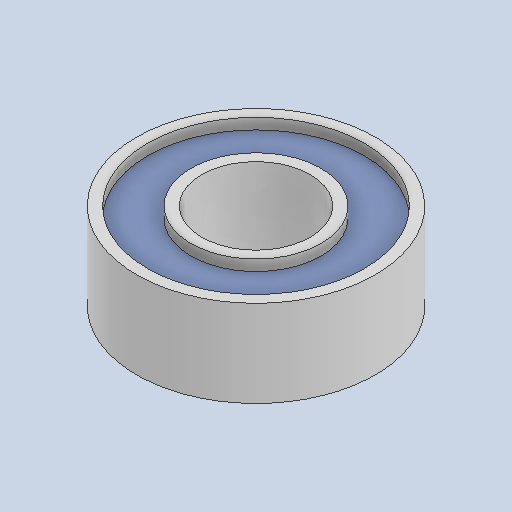
# Autodesk Inventor part: Bearing_5x11x4
Saved by Autodesk Inventor 2022 (Build 260153000, 153)
## iProperties
Created: 2021-06-16
Part Number: Bearing_5x11x4
Material: Generic
Document SubType Name: Modeling
Designer: burgessb
Density: 1 g/cm^3
Appearance: Default
Author: burgessb
Autodesk Inventor part; units mm, degrees
ref_plane "YZ Plane" through (0, 0, 0) normal (1, 0, 0) x (0, 1, 0)
ref_plane "XZ Plane" through (0, 0, 0) normal (0, 1, 0) x (-1, 0, 0)
ref_plane "XY Plane" through (0, 0, 0) normal (0, 0, 1) x (1, 0, 0)
sketch "Sketch1" plane through (0, 0, 0) normal (0, 1, 0) x (-1, 0, 0)
  circle A0 centre (0, 0) radius 5.5
  circle A1 centre (0, 0) radius 2.5
  dimension "d0" = 11
  dimension "d1" = 5
  constraints: 2 centre point, 2 coincident
  measures "d0" diameter of A0
  measures "d1" diameter of A1
extrude "Extrusion1" add sketch "Sketch1" along normal blind 4
sketch "Sketch2" plane through (0, 4, 0) normal (0, 1, 0) x (1, 0, 0)
  circle A0 centre (0, 0) radius 5.5 projected
  circle A1 centre (0, 0) radius 2.5 projected
  circle A2 centre (0, 0) radius 3
  circle A3 centre (0, 0) radius 5
  dimension "d4" = 0.5
  dimension "d5" = 0.5
  constraints: 2 centre point
  measures "d4" radial gap between concentric circles of A1 A2
  measures "d5" radial gap between concentric circles of A0 A3
extrude "Extrusion2" cut sketch "Sketch2" against normal blind 0.5 contours A3
sketch "Sketch3" plane through (0, 0, 0) normal (0, -1, 0) x (1, 0, 0)
  circle A0 centre (0, 0) radius 5.5 projected
  circle A1 centre (0, 0) radius 2.5 projected
  circle A2 centre (0, 0) radius 5 projected
  circle A3 centre (0, 0) radius 3 projected
extrude "Extrusion3" cut sketch "Sketch3" against normal blind 0.5 contours A2
body "Solid1"
